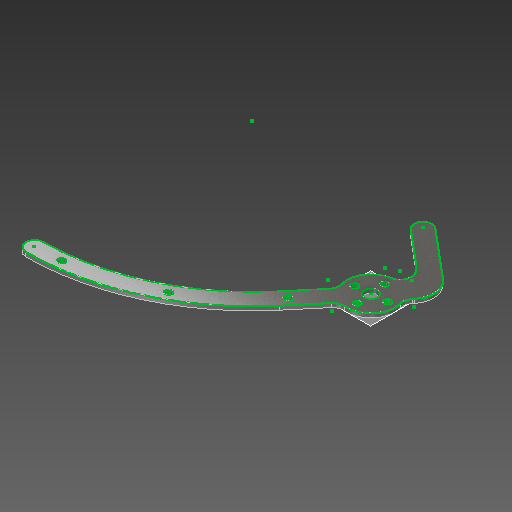
# Autodesk Inventor part: wstepna_geometria_wersja_2
Saved by Autodesk Inventor 2022 (Build 260153000, 153)
## iProperties
Created: 2022-02-09
Part Number: wstepna_geometria_wersja_2
Material: Generic
Document SubType Name: Modeling
Designer: Tomasz Krakowski
Density: 1 g/cm^3
Appearance: Honowane
Author: Tomasz Krakowski
Autodesk Inventor part; units mm, degrees
ref_plane "YZ Plane" through (0, 0, 0) normal (1, 0, 0) x (0, 1, 0)
ref_plane "XZ Plane" through (0, 0, 0) normal (0, 1, 0) x (-1, 0, 0)
ref_plane "XY Plane" through (0, 0, 0) normal (0, 0, 1) x (1, 0, 0)
ref_plane "Work Plane5" through (0, 3, 0) normal (0, 1, 0) x (1, 0, 0)
sketch "Sketch2" plane through (0, 3, 0) normal (0, 1, 0) x (1, 0, 0)
  line L0 (0, 0) -> (-19.2836, -22.9813) construction
  line L1 (5.1953, 21.7488) -> (-13.9558, 37.8185) construction
  arc A0 (-95.8881, -58.7026) -> (-19.2836, -22.9813) centre (-95.8881, 41.2974) ccw construction
  line L2 (-19.2836, -22.9813) -> (-95.8881, 41.2974) construction
  line L3 (-95.8881, 41.2974) -> (-95.8881, -58.7026) construction
  line L4 (0, 0) -> (0, -11) construction
  line L5 (6.4279, 7.6604) -> (0, 0) construction
  arc A1 (6.4279, 7.6604) -> (5.1953, 21.7488) centre (-1.2326, 14.0883) ccw construction
  arc A2 (-95.8881, -54.7026) -> (-95.8881, -62.7026) centre (-95.8881, -58.7026) ccw
  arc A3 (-95.8881, -62.7026) -> (-16.2195, -25.5525) centre (-95.8881, 41.2974) ccw
  arc A4 (-95.8881, -54.7026) -> (-22.3478, -20.4102) centre (-95.8881, 41.2974) ccw
  line L6 (-19.2836, -22.9813) -> (-22.3478, -20.4102) construction
  line L7 (-19.2836, -22.9813) -> (-16.2195, -25.5525) construction
  line L8 (10.8306, 22.2418) -> (-11.3847, 40.8826)
  arc A5 (-11.3847, 40.8826) -> (-16.527, 34.7543) centre (-13.9558, 37.8185) ccw
  line L9 (-0.44, 21.2557) -> (-16.527, 34.7543)
  arc A6 (2.0873, 18.0456) -> (-0.44, 21.2557) centre (-6.8679, 13.5953) ccw
  arc A7 (12.0632, 8.1535) -> (10.8306, 22.2418) centre (4.4028, 14.5813) ccw
  circle A8 centre (0, 0) radius 7 construction
  arc A9 (-1.1061, -10.9442) -> (10.5859, 2.9897) centre (0, 0) ccw
  arc A10 (-1.6433, 10.8766) -> (-10.5859, -2.9897) centre (0, 0) ccw
  line L10 (-16.2195, -25.5525) -> (-5.4391, -12.705)
  line L11 (11.5675, 7.5627) -> (12.0632, 8.1535)
  line L12 (-22.3478, -20.4102) -> (-11.5675, -7.5627)
  arc A11 (-1.1061, -10.9442) -> (-5.4391, -12.705) centre (-1.6089, -15.9189) ccw
  arc A12 (11.5675, 7.5627) -> (10.5859, 2.9897) centre (15.3977, 4.3487) ccw
  arc A13 (-11.5675, -7.5627) -> (-10.5859, -2.9897) centre (-15.3977, -4.3487) ccw
  arc A14 (-1.6433, 10.8766) -> (2.0873, 18.0456) centre (-2.3903, 15.8204) ccw
  circle A15 centre (0, 0) radius 3
  circle A16 centre (-6.9734, -0.6101) radius 1.5
  line L13 (0, 0) -> (-6.9734, -0.6101) construction
  circle A17 centre (0.6101, -6.9734) radius 1.5
  circle A18 centre (6.9734, 0.6101) radius 1.5
  circle A19 centre (-0.6101, 6.9734) radius 1.5
  point P0 (12.8558, 15.3209)
  point P1 (-3.5224, -10.4208)
  point P2 (9.6508, 5.2785)
  dimension "d53" = 14
  dimension "d24" = 30
  dimension "d27" = 35
  dimension "d28" = 20
  dimension "d29" = 100
  dimension "d30" = 50
  dimension "d41" = 10
  dimension "d42" = 140
  dimension "d50" = 8
  dimension "d51" = 4
  dimension "d52" = 10
  dimension "d55" = 11
  dimension "d56" = 11
  dimension "d57" = 5
  dimension "d58" = 6
  dimension "d62" = 3
  dimension "d63" = 45
  dimension "d66" = 360
  constraints: 31 point on circle, 28 end point, 23 tangent, 19 centre point, 8 coincident, 5 perpendicular, 4 equal radius, 4 point on line, 2 collinear, 1 vertical, 12 other
  measures "d24" distance of L0.start L0.end
  measures "d27" distance of point (12.856, 15.321) L1.end
  measures "d28" distance of point (12.856, 15.321) L0.start
  measures "d29" radius of A0
  measures "d30" angle of L3 L2
  measures "d41" radius of A1
  measures "d42" angle of L4 L0
  measures "d50" diameter of A2
  measures "d51" radius of A5
  measures "d52" radius of A6
  measures "d55" radius of A10
  measures "d56" radius of A9
  measures "d57" radius of A11
  measures "d58" diameter of A15
  measures "d62" diameter of A16
  measures "d63" angle of L0 L13
extrude "Extrusion2" add sketch "Sketch2" along normal blind 2
sketch "Sketch4" plane through (0, 5, 0) normal (0, 1, 0) x (1, 0, 0)
  arc A0 (-95.8881, -54.7026) -> (-22.3478, -20.4102) centre (-95.8881, 41.2974) ccw construction
  arc A1 (-84.2223, -58.0198) -> (-17.4113, -20.6815) centre (-95.8881, 41.2974) ccw construction
  line L0 (-84.2223, -58.0198) -> (-95.8881, 41.2974) construction
  line L1 (-95.8881, 41.2974) -> (-17.4113, -20.6815) construction
  circle A2 centre (0, 0) radius 3 construction
  line L2 (-95.8881, 41.2974) -> (0, 0) construction
  point P0 (-47.1033, -45.9954)
  dimension "d68" = 4
  dimension "d69" = 45
  dimension "d70" = 15
  constraints: 6 end point, 4 coincident, 3 point on circle, 1 centre point
  measures "d68" radial gap between concentric circles of A0 A1
  measures "d69" angle of L1 L0
  measures "d70" angle of L2 L1
hole "Hole1" at (-84.2223, 5, 58.0198) at (-47.1033, 5, 45.9954) at (-17.4113, 5, 20.6815) direction (0, -1, 0) diameter 3.2 end through all
sketch "Sketch5" plane through (0, 5, 0) normal (0, 1, 0) x (1, 0, 0)
  circle A0 centre (-47.1033, -45.9954) radius 1.6 projected
  circle A1 centre (-84.2223, -58.0198) radius 1.6 projected
  circle A2 centre (-17.4113, -20.6815) radius 1.6 projected
  circle A3 centre (0, 0) radius 3 projected
  circle A4 centre (-0.6101, 6.9734) radius 1.5 projected
  circle A5 centre (6.9734, 0.6101) radius 1.5 projected
  circle A6 centre (0.6101, -6.9734) radius 1.5 projected
  circle A7 centre (-6.9734, -0.6101) radius 1.5 projected
  arc A8 (-95.8881, -62.7026) -> (-16.2195, -25.5525) centre (-95.8881, 41.2974) ccw projected
  line L0 (-16.2195, -25.5525) -> (-5.4391, -12.705) projected
  arc A9 (-1.1061, -10.9442) -> (-5.4391, -12.705) centre (-1.6089, -15.9189) ccw projected
  arc A10 (-1.1061, -10.9442) -> (10.5859, 2.9897) centre (0, 0) ccw projected
  arc A11 (11.5675, 7.5627) -> (10.5859, 2.9897) centre (15.3977, 4.3487) ccw projected
  line L1 (11.5675, 7.5627) -> (12.0632, 8.1535) projected
  arc A12 (12.0632, 8.1535) -> (10.8306, 22.2418) centre (4.4028, 14.5813) ccw projected
  line L2 (10.8306, 22.2418) -> (-11.3847, 40.8826) projected
  arc A13 (-11.3847, 40.8826) -> (-16.527, 34.7543) centre (-13.9558, 37.8185) ccw projected
  line L3 (-16.527, 34.7543) -> (-0.44, 21.2557) projected
  arc A14 (2.0873, 18.0456) -> (-0.44, 21.2557) centre (-6.8679, 13.5953) ccw projected
  arc A15 (-1.6433, 10.8766) -> (2.0873, 18.0456) centre (-2.3903, 15.8204) ccw projected
  arc A16 (-1.6433, 10.8766) -> (-10.5859, -2.9897) centre (0, 0) ccw projected
  arc A17 (-11.5675, -7.5627) -> (-10.5859, -2.9897) centre (-15.3977, -4.3487) ccw projected
  line L4 (-11.5675, -7.5627) -> (-22.3478, -20.4102) projected
  arc A18 (-95.8881, -54.7026) -> (-22.3478, -20.4102) centre (-95.8881, 41.2974) ccw projected
  arc A19 (-95.8881, -54.7026) -> (-95.8881, -62.7026) centre (-95.8881, -58.7026) ccw projected
body "Solid2"
